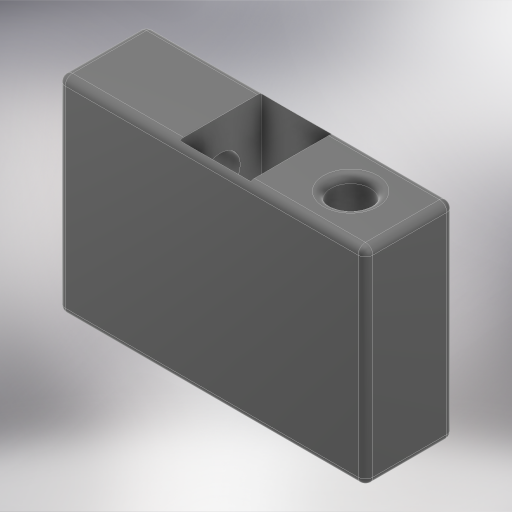
# Autodesk Inventor part: .5x1 Tube Stock Insert
Saved by Autodesk Inventor 2024 (Build 280153000, 153)
## iProperties
Created: 2023-12-17
Part Number: .5x1 Tube Stock Insert
Material: PBT Plastic
Document SubType Name: Modeling
Designer: aaron
Density: 1.31 g/cm^3
Appearance: Smooth - White
Author: aaron
Autodesk Inventor part; units mm, degrees
ref_plane "YZ Plane" through (0, 0, 0) normal (1, 0, 0) x (0, 1, 0)
ref_plane "XZ Plane" through (0, 0, 0) normal (0, 1, 0) x (-1, 0, 0)
ref_plane "XY Plane" through (0, 0, 0) normal (0, 0, 1) x (1, 0, 0)
sketch "Sketch1" plane through (0, 0, 0) normal (1, 0, 0) x (0, 1, 0)
  line L0 (-11.1125, -4.7625) -> (11.1125, -4.7625)
  line L1 (11.1125, -4.7625) -> (11.1125, 4.7625)
  line L2 (11.1125, 4.7625) -> (-11.1125, 4.7625)
  line L3 (-11.1125, 4.7625) -> (-11.1125, -4.7625)
  line L4 (-11.1125, -4.7625) -> (11.1125, 4.7625) construction
  line L5 (11.1125, -4.7625) -> (-11.1125, 4.7625) construction
  circle A0 centre (5.5563, 0) radius 2.1082
  circle A1 centre (-5.5562, 0) radius 2.1082
  point P0 (0, 0)
  point P1 (-11.1125, 0)
  dimension "d0" = 9.525
  dimension "d1" = 22.225
  dimension "d2" = 4.2164
  dimension "d3" = 4.2164
  dimension "d4" = 5.5563
  dimension "d5" = 5.5563
  constraints: 12 end point, 3 midpoint, 2 centre point, 2 parallel, 1 horizontal, 1 perpendicular
  measures "d0" distance between parallel lines of L2 L0
  measures "d1" distance from line of point (-11.112, 0) L1
  measures "d2" diameter of A0
  measures "d3" diameter of A1
  measures "d4" distance from line of L3 A1.centre
  measures "d5" distance from line of L1 A0.centre
extrude "Extrusion1" add sketch "Sketch1" along normal blind 12.7
sketch "Sketch2" plane through (12.7, 0, 0) normal (1, 0, 0) x (0, 0, -1)
  circle A0 centre (0, 5.5563) radius 2.1082 projected
  line L0 (0, 10.5972) -> (4.3656, 8.0767)
  line L1 (4.3656, 8.0767) -> (4.3656, 3.0358)
  line L2 (4.3656, 3.0358) -> (0, 0.5153)
  line L3 (0, 0.5153) -> (-4.3656, 3.0358)
  line L4 (-4.3656, 3.0358) -> (-4.3656, 8.0767)
  line L5 (-4.3656, 8.0767) -> (0, 10.5972)
  circle A1 centre (0, -5.5562) radius 2.1082 projected
  line L6 (0, -0.5153) -> (4.3656, -3.0358)
  line L7 (4.3656, -3.0358) -> (4.3656, -8.0767)
  line L8 (4.3656, -8.0767) -> (0, -10.5972)
  line L9 (0, -10.5972) -> (-4.3656, -8.0767)
  line L10 (-4.3656, -8.0767) -> (-4.3656, -3.0358)
  line L11 (-4.3656, -3.0358) -> (0, -0.5153)
  line L12 (4.7625, 11.1125) -> (-4.7625, 11.1125) projected
  line L13 (-4.7625, 11.1125) -> (-4.7625, -11.1125) projected
  line L14 (-4.7625, -11.1125) -> (4.7625, -11.1125) projected
  line L15 (4.7625, -11.1125) -> (4.7625, 11.1125) projected
  circle A2 centre (0, 5.5563) radius 2.1082 projected
  circle A3 centre (0, -5.5562) radius 2.1082 projected
  line L16 (-4.3656, 8.0767) -> (4.3656, 8.0767)
  line L17 (4.3656, 8.0767) -> (4.3656, 13.7838)
  line L18 (4.3656, 13.7838) -> (-4.3656, 13.7838)
  line L19 (-4.3656, 13.7838) -> (-4.3656, 8.0767)
  line L20 (-4.3656, -8.0767) -> (4.3656, -8.0767)
  line L21 (4.3656, -8.0767) -> (4.3656, -13.1177)
  line L22 (4.3656, -13.1177) -> (-4.3656, -13.1177)
  line L23 (-4.3656, -13.1177) -> (-4.3656, -8.0767)
  point P0 (-4.3656, 11.1125)
  point P1 (-4.3656, -11.1125)
  point P2 (4.3656, -11.1125)
  point P3 (4.3656, 11.1125)
  dimension "d10" = 4.3656
  dimension "d11" = 4.3656
  constraints: 40 end point, 4 parallel, 2 coincident, 2 horizontal, 2 perpendicular, 2 point on line, 26 other
  measures "d10" distance from line of L1 point (0, 5.556)
  measures "d11" distance from line of L7 point (0, -5.556)
extrude "Extrusion2" add sketch "Sketch2" along normal blind 7.62 contours L17 L12 L15 L14 L21 L7 L6 L11 L10 L23 L13 L19 L4 L3 L2 L1
sketch "Sketch3" plane through (20.32, 0, 0) normal (1, 0, 0) x (0, 0, -1)
  line L0 (-4.7625, 11.1125) -> (-4.7625, -11.1125) projected
  line L1 (4.7625, -11.1125) -> (-4.7625, -11.1125)
  line L2 (-4.7625, -11.1125) -> (-4.7625, 11.1125)
  line L3 (-4.7625, 11.1125) -> (4.7625, 11.1125)
  line L4 (4.7625, 11.1125) -> (4.7625, -11.1125)
  line L5 (4.7625, -11.1125) -> (-4.7625, 11.1125) construction
  line L6 (-4.7625, -11.1125) -> (4.7625, 11.1125) construction
  point P0 (0, 0)
  constraints: 12 end point, 2 midpoint, 2 parallel, 1 horizontal, 1 perpendicular
extrude "Extrusion3" add sketch "Sketch3" along normal blind 12.7
sketch "Sketch4" plane through (0, 11.1125, 4.7625) normal (0, 1, 0) x (1, 0, 0)
  circle A0 centre (26.67, 4.7625) radius 2.1082
  line L0 (33.02, 9.525) -> (33.02, 0) projected
  point P0 (0, 4.7625)
  dimension "d16" = 4.2164
  dimension "d17" = 6.35
  constraints: 1 centre point
  measures "d16" diameter of A0
  measures "d17" distance from line of L0 A0.centre
extrude "Extrusion4" cut sketch "Sketch4" against normal blind 25.4
fillet "Fillet1" radius 0.7937 4 edges at (33.02, 0, -4.7625) (33.02, 11.1125, 0) (33.02, 0, 4.7625) (33.02, -11.1125, 0)
fillet "Fillet2" radius 0.7937 8 edges at (32.7875, 10.88, -4.53) (16.1131, 11.1125, -4.7625) (32.7875, 10.88, 4.53) (16.1131, 11.1125, 4.7625) (32.7875, -10.88, -4.53) (16.1131, -11.1125, -4.7625) (32.7875, -10.88, 4.53) (16.1131, -11.1125, 4.7625)
fillet "Fillet3" radius 0.7937 8 edges at (0, 10.88, 4.53) (0, 0, 4.7625) (0, -10.88, 4.53) (0, -11.1125, 0) (0, -10.88, -4.53) (0, 0, -4.7625) (0, 10.88, -4.53) (0, 11.1125, 0)
fillet "Fillet4" radius 0.7937 2 edges at (24.5618, 11.1125, 0) (24.5618, -11.1125, 0)
fillet "Fillet5" radius 0.3969 2 edges at (0, 3.4481, 0) (0, -7.6644, 0)
body "Solid1"
